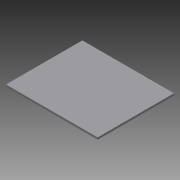
# Autodesk Inventor part: Part9
Saved by Autodesk Inventor 2015 (Build 190159000, 159)
## iProperties
Created: 2015-07-12
Part Number: Part9
Material: Generic
Document SubType Name: Modeling
Designer: tsayman
Density: 1 g/cm^3
Appearance: Default
Author: tsayman
Autodesk Inventor part; units mm, degrees
ref_plane "YZ Plane" through (0, 0, 0) normal (1, 0, 0) x (0, 1, 0)
ref_plane "XZ Plane" through (0, 0, 0) normal (0, 1, 0) x (-1, 0, 0)
ref_plane "XY Plane" through (0, 0, 0) normal (0, 0, 1) x (1, 0, 0)
sketch "Sketch1" plane through (0, 0, 0) normal (0, 1, 0) x (-1, 0, 0)
  line L0 (-12.7, -1435.0315) -> (292.1, -1435.0315)
  line L1 (292.1, -1435.0315) -> (292.1, -1689.0315)
  line L2 (292.1, -1689.0315) -> (-12.7, -1689.0315)
  line L3 (-12.7, -1689.0315) -> (-12.7, -1435.0315)
  line L4 (0, 0) -> (-304.8, 0)
  line L5 (-304.8, 0) -> (-304.8, -254)
  line L6 (-304.8, -254) -> (0, -254)
  line L7 (0, -254) -> (0, 0)
  dimension "d0" = 304.8
  dimension "d1" = 254
  dimension "d2" = 304.8
  dimension "d3" = 254
  constraints: 16 end point, 4 parallel, 2 horizontal, 2 perpendicular
  measures "d0" distance of L1.end L2.end
  measures "d1" distance of L0.end L1.end
  measures "d2" distance of L6.end L5.end
  measures "d3" distance of L5.end L4.end
extrude "Extrusion1" add sketch "Sketch1" along normal blind 6.35 contours L7 L6 L5 L4
body "Solid1"
